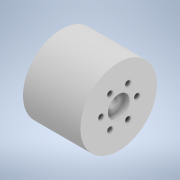
# Autodesk Inventor part: rcr-S3
Saved by Autodesk Inventor 2022 (Build 260153000, 153)
## iProperties
Created: 2022-02-21
Part Number: rcr-S3
Material: Generic
Document SubType Name: Modeling
Designer: olivi
Density: 1 g/cm^3
Appearance: Default
Author: olivi
Autodesk Inventor part; units mm, degrees
ref_plane "YZ Plane" through (0, 0, 0) normal (1, 0, 0) x (0, 1, 0)
ref_plane "XZ Plane" through (0, 0, 0) normal (0, 1, 0) x (-1, 0, 0)
ref_plane "XY Plane" through (0, 0, 0) normal (0, 0, 1) x (1, 0, 0)
sketch "Sketch4" plane through (0, 0, 0) normal (1, 0, 0) x (0, 1, 0)
  circle A0 centre (0, 0) radius 50.8
  circle A1 centre (0, 0) radius 6.35
  circle A2 centre (0, -23.8252) radius 3.4336
  circle A3 centre (20.6332, -11.9126) radius 3.4336
  circle A4 centre (0, 0) radius 6.35
  circle A5 centre (20.6332, 11.9126) radius 3.4336
  circle A6 centre (0, 0) radius 6.35
  circle A7 centre (0, 23.8252) radius 3.4336
  circle A8 centre (0, 0) radius 6.35
  circle A9 centre (-20.6332, 11.9126) radius 3.4336
  circle A10 centre (0, 0) radius 6.35
  circle A11 centre (-20.6332, -11.9126) radius 3.4336
  circle A12 centre (0, 0) radius 6.35
  dimension "d12" = 101.6
  dimension "d13" = 12.7
  dimension "d14" = 23.8252
  dimension "d17" = 360
  constraints: 13 centre point, 4 coincident, 23 other
  measures "d12" diameter of A0
  measures "d13" diameter of A1
  measures "d14" distance of point (0, 0) A2.centre
extrude "Extrusion3" add sketch "Sketch4" along normal blind 76.2
sketch "Sketch5" plane through (76.2, 0, 0) normal (1, 0, 0) x (0, 0, -1)
  circle A0 centre (0, 0) radius 6.35 projected
  circle A1 centre (0, 0) radius 14.2875
  dimension "d21" = 28.575
  constraints: 1 centre point, 1 coincident
  measures "d21" diameter of A1
extrude "Extrusion4" cut sketch "Sketch5" against normal blind 8.001
body "Solid2"
